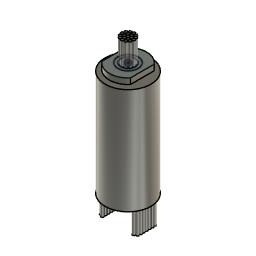
LMP-30A v1 (Autodesk Fusion 360 design; units mm, degrees)
Autodesk Fusion 360 part; units mm, degrees
note: some values were not read from the file. Chosen so that the rebuilt part matches the saved one: which bodies a step acts on.
sketch "Sketch1" plane through (0, 0, 0) normal (0, 0, 1) x (1, 0, 0)
  circle A0 centre (0, 0) radius 8
  dimension "d1" = 16
  constraint coincident A0.centre origin
  measures "d1" diameter of A0
extrude "Extrude1" add sketch "Sketch1" along normal blind 37 makes body 1
sketch "Sketch2" plane through (0, 0, 37) normal (0, 0, 1) x (-1, 0, 0)
  circle A0 centre (0, 0) radius 8
  circle A1 centre (0, 0) radius 3.5
  dimension "d4" = 7
  constraint concentric A0 A1
  measures "d4" diameter of A1
extrude "Extrude2" add sketch "Sketch2" along normal blind 0.5 contours A1 bodies 1
sketch "Sketch3" plane through (0, 0, 37.5) normal (0, 0, 1) x (-1, 0, 0)
  circle A0 centre (0, 0) radius 3.5
  circle A1 centre (0, 0) radius 6.5
  line L0 (5, 6.5) -> (-5, 6.5)
  line L1 (-5, 6.5) -> (-5, -6.5)
  line L2 (-5, -6.5) -> (5, -6.5)
  line L3 (5, -6.5) -> (5, 6.5)
  dimension "d7" = 13
  dimension "d8" = 13
  constraint concentric A0 A1
  constraint horizontal L0
  constraint vertical L1
  constraint horizontal L2
  constraint vertical L3
  measures "d7" diameter of A1
  measures "d8" distance of L0.start L2.end
extrude "Extrude3" add sketch "Sketch3" along normal blind 2 contours A0 | A1 L1 L3 bodies 1
sketch "Sketch4" plane through (0, 0, 39.5) normal (0, 0, 1) x (-1, 0, 0)
  arc A0 (-5, -4.1533) -> (5, -4.1533) centre (0, 0) ccw
  line L0 (5, -4.1533) -> (5, 4.1533)
  arc A1 (5, 4.1533) -> (-5, 4.1533) centre (0, 0) ccw
  line L1 (-5, 4.1533) -> (-5, -4.1533)
  circle A2 centre (0, 0) radius 3.5
  dimension "d11" = 7
  constraint concentric A0 A2
  measures "d11" diameter of A2
sketch "Sketch5" plane through (0, 0, 39.5) normal (0, 0, 1) x (-1, 0, 0)
  circle A0 centre (0, 0) radius 2.5
  dimension "d12" = 5
  constraint coincident A0.centre origin
  measures "d12" diameter of A0
sketch "Sketch7" plane through (0, 0, 39.5) normal (0, 0, 1) x (-1, 0, 0)
  circle A0 centre (0, 2) radius 0.5
  dimension "d13" = 1
  measures "d13" diameter of A0
extrude "Extrude4" add sketch "Sketch7" along normal blind 8 bodies 1
pattern_circular "C-Pattern1" count 12 over 360 about axis through (0, 0, 1.75) along (0, 0, 1) of "Extrude4"
sketch "Sketch8" plane through (0, 0, 39.5) normal (0, 0, 1) x (-1, 0, 0)
  circle A0 centre (-0.75, 0.75) radius 0.5
  dimension "d18" = 1
  measures "d18" diameter of A0
extrude "Extrude5" add sketch "Sketch8" along normal blind 8 bodies 1
pattern_circular "C-Pattern2" count 6 over 360 about axis through (0, 0, 1.75) along (0, 0, 1) of "Extrude5"
sketch "Sketch9" plane through (0, 0, 39.5) normal (0, 0, 1) x (-1, 0, 0)
  circle A0 centre (0, 0) radius 0.5
  dimension "d23" = 1
  constraint coincident A0.centre origin
  measures "d23" diameter of A0
extrude "Extrude6" add sketch "Sketch9" along normal blind 8 bodies 1
sketch "Sketch10" plane through (0, 0, 0) normal (0, 0, -1) x (1, 0, 0)
  circle A0 centre (0, 0) radius 8
  circle A1 centre (0, 0) radius 7.5
  line L0 (-5.5902, -5) -> (5.5902, -5)
  line L1 (-5.5902, 5) -> (5.5902, 5)
  line L2 (-5.5902, -5) -> (-5.5902, 5)
  line L3 (5.5902, -5) -> (5.5902, 5)
  dimension "d26" = 15
  constraint concentric A0 A1
  constraint horizontal L0
  constraint horizontal L1
  constraint coincident A1 L0.start
  constraint coincident A1 L0.end
  constraint coincident A1 L1.start
  constraint coincident A1 L1.end
  constraint vertical L2
  constraint coincident L0.start L2.start
  constraint coincident L1.start L2.end
  constraint vertical L3
  constraint coincident L0.end L3.start
  constraint coincident L1.end L3.end
  measures "d26" diameter of A1
sketch "Sketch12" plane through (0, 0, 0) normal (0, 0, -1) x (1, 0, 0)
  line L0 (-5, -4) -> (-5.5902, -4)
  line L1 (-5, -4) -> (-5, 4)
  line L2 (-5, 4) -> (-5.5902, 4)
  line L3 (-5.5902, -5) -> (-5.5902, 5)
  line L4 (5, 4) -> (5.5902, 4)
  line L5 (5, 4) -> (5, -4)
  line L6 (5, -4) -> (5.5902, -4)
  line L7 (5.5902, -5) -> (5.5902, 5)
  dimension "d29" = 10
  constraint horizontal L0
  constraint perpendicular L0 L1
  constraint perpendicular L1 L2
  constraint coincident L0.end L3
  constraint horizontal L4
  constraint perpendicular L4 L5
  constraint perpendicular L5 L6
  constraint coincident L4.end L7
  constraint equal L2 L4
  constraint coincident L2.end L3
  measures "d29" distance of L1 L5
extrude "Extrude7" cut sketch "Sketch12" sketch "Sketch10" against normal blind 2 of sketch 2 contours A1 L3 | A1 L2 bodies 1
sketch "Sketch13" plane through (0, 0, 2) normal (0, 0, -1) x (1, 0, 0)
  line L0 (-5, 4) -> (-5.5902, 4)
  line L1 (-5.5902, 4) -> (-5.5902, 5)
  arc A0 (-5.5902, 5) -> (-5.5902, -5) centre (0, 0) ccw
  line L2 (-5.5902, -5) -> (-5.5902, -4)
  line L3 (-5.5902, -4) -> (-5, -4)
  line L4 (-5, -4) -> (-5, 4)
  circle A1 centre (-5.5, 3.5) radius 0.5
  circle A2 centre (-5.5, 2.5) radius 0.5
  circle A3 centre (-5.5, 1.5) radius 0.5
  circle A4 centre (-5.5, 0.5) radius 0.5
  circle A5 centre (-5.5, -0.5) radius 0.5
  circle A6 centre (-5.5, -1.5) radius 0.5
  circle A7 centre (-5.5, -2.5) radius 0.5
  circle A8 centre (-5.5, -3.5) radius 0.5
  circle A9 centre (-6.345, -3) radius 0.475
  circle A10 centre (-6.4, -2) radius 0.5
  circle A11 centre (-6.4, -1) radius 0.5
  circle A12 centre (-6.4, 0) radius 0.5
  circle A13 centre (-6.4, 1) radius 0.5
  circle A14 centre (-6.4, 2) radius 0.5
  circle A15 centre (-6.345, 3) radius 0.475
  circle A16 centre (5.5, -3.5) radius 0.5
  circle A17 centre (5.5, -2.5) radius 0.5
  circle A18 centre (5.5, -1.5) radius 0.5
  circle A19 centre (5.5, -0.5) radius 0.5
  circle A20 centre (5.5, 0.5) radius 0.5
  circle A21 centre (5.5, 1.5) radius 0.5
  circle A22 centre (5.5, 2.5) radius 0.5
  circle A23 centre (5.5, 3.5) radius 0.5
  circle A24 centre (6.4, 2) radius 0.5
  circle A25 centre (6.4, 1) radius 0.5
  circle A26 centre (6.4, 0) radius 0.5
  circle A27 centre (6.4, -1) radius 0.5
  circle A28 centre (6.4, -2) radius 0.5
  circle A29 centre (6.34, -3) radius 0.475
  circle A30 centre (6.34, 3) radius 0.475
  dimension "d32" = 1
  dimension "d33" = 1
  dimension "d34" = 1
  dimension "d35" = 1
  dimension "d36" = 1
  dimension "d37" = 1
  dimension "d38" = 1
  dimension "d39" = 1
  dimension "d40" = 0.95
  dimension "d41" = 1
  dimension "d42" = 1
  dimension "d43" = 1
  dimension "d44" = 1
  dimension "d45" = 1
  dimension "d46" = 0.95
  dimension "d47" = 1
  dimension "d48" = 1
  dimension "d49" = 1
  dimension "d50" = 1
  dimension "d51" = 1
  dimension "d52" = 1
  dimension "d53" = 1
  dimension "d54" = 1
  dimension "d55" = 1
  dimension "d56" = 1
  dimension "d57" = 1
  dimension "d58" = 1
  dimension "d59" = 1
  dimension "d60" = 0.95
  dimension "d61" = 0.95
  measures "d32" diameter of A1
  measures "d33" diameter of A2
  measures "d34" diameter of A3
  measures "d35" diameter of A4
  measures "d36" diameter of A5
  measures "d37" diameter of A6
  measures "d38" diameter of A7
  measures "d39" diameter of A8
  measures "d40" diameter of A9
  measures "d41" diameter of A10
  measures "d42" diameter of A11
  measures "d43" diameter of A12
  measures "d44" diameter of A13
  measures "d45" diameter of A14
  measures "d46" diameter of A15
  measures "d47" diameter of A16
  measures "d48" diameter of A17
  measures "d49" diameter of A18
  measures "d50" diameter of A19
  measures "d51" diameter of A20
  measures "d52" diameter of A21
  measures "d53" diameter of A22
  measures "d54" diameter of A23
  measures "d55" diameter of A24
  measures "d56" diameter of A25
  measures "d57" diameter of A26
  measures "d58" diameter of A27
  measures "d59" diameter of A28
  measures "d60" diameter of A29
  measures "d61" diameter of A30
extrude "Extrude8" add sketch "Sketch13" along normal blind 10 separate body contours A1 | A2 | A3 | A4 | A5 | A8 | A6 | A7 | A9 | A10 | A14 | A13 | A12 | A11 | A15 | A16 | A23 | A22 | A21 | A20 | A19 | A18 | A17 | A24 | A28 | A27 | A26 | A25 | A29 | A30 makes body 7 at (-5.5249, -3.9994, -1.3333) makes body 7 at (-5.0442, -2.2944, -1.3333) makes body 7 at (-5.08, -1.2287, -4.6667) makes body 7 at (-5.1421, -0.8491, -4.6667) makes body 7 at (-5.1786, 0.883, -4.6667) makes body 7 at (-5.1421, 1.8491, -4.6667) makes body 7 at (-5.1981, 2.8986, -4.6667) makes body 7 at (-5.5249, 3.9994, -4.6667) makes body 3 at (-5.9711, -2.2571, -4.6667) makes body 3 at (-6.0421, -1.3491, -4.6667) makes body 3 at (-6.0421, 0.3491, -4.6667) makes body 3 at (-6.0786, 1.383, -1.3333) makes body 3 at (-6.3266, 2.4946, -4.6667) makes body 2 at (5.0843, 3.2222, -4.6667) makes body 2 at (5.9558, 2.7056, -1.3333) makes body 2 at (5.8579, 1.8491, -4.6667) makes body 2 at (5.92, 0.7713, -4.6667) makes body 2 at (5.8579, -0.1509, -4.6667) makes body 2 at (5.8214, -1.117, -4.6667) makes body 2 at (5.8579, -2.1509, -4.6667) makes body 2 at (5.4025, -3.0096, -4.6667) makes body 6 at (6.2785, 1.515, -4.6667) makes body 6 at (6.7579, 0.6509, -4.6667) makes body 6 at (6.7214, -0.383, -1.3333) makes body 6 at (6.7579, -0.6509, -4.6667) makes body 6 at (6.3025, -1.5096, -4.6667) makes body 8 at (-5.8706, -2.9763, -4.6667) makes body 9 at (-5.8706, 3.0237, -4.6667) makes body 4 at (6.8144, 3.0237, -4.6667) makes body 5 at (6.8144, -2.9763, -4.6667)
